Cale Nema14 (Autodesk Fusion 360 design; units mm, degrees)
Autodesk Fusion 360 part; units mm, degrees
sketch "Sketch1" plane through (0, 0, 0) normal (0, 0, 1) x (1, 0, 0)
  line L0 (24, 0) -> (24, 11) construction
  line L1 (-24, 11) -> (-24, 0) construction
  arc A0 (20.9184, 45.8497) -> (-20.9184, 45.8497) centre (0, 44) ccw construction
  line L2 (24, 11) -> (-24, 11) construction
  line L3 (-24, 0) -> (24, 0) construction
  line L4 (0, 44) -> (0, 11) construction
  line L5 (-24.1506, 0) -> (-24.1506, 11)
  line L6 (24.1506, 0) -> (24.1506, 11)
  line L7 (-23.1779, 22) -> (23.1779, 22)
  line L8 (-23.1779, 22) -> (-24.1506, 11)
  line L9 (24.1506, 11) -> (23.1779, 22)
  line L10 (24, 11) -> (20.9184, 45.8497) construction
  line L11 (-24, 11) -> (-20.9184, 45.8497) construction
  line L12 (-24.1506, 0) -> (24.1506, 0)
  line L13 (24, 0) -> (27, 0)
  line L14 (27, 0) -> (27, 22)
  line L15 (23.1779, 22) -> (27, 22)
  line L16 (-23.1779, 22) -> (-27, 22)
  line L17 (-27, 22) -> (-27, 0)
  line L18 (-27, 0) -> (-24, 0)
  dimension "d1" = 48
  dimension "d2" = 11
  dimension "d3" = 21
  dimension "d5" = 33
  dimension "d6" = 11
  dimension "d8" = 11
  dimension "d9" = 11
  dimension "d10" = 11
  dimension "d12" = 0.15
  dimension "d13" = 0.15
  dimension "d14" = 3
  dimension "d15" = 3
  constraint perpendicular L0 L3
  constraint perpendicular L0 L2
  constraint perpendicular L1 L2
  constraint coincident A0.centre L4.start
  constraint midpoint L2 L4.end
  constraint perpendicular L2 L4
  constraint horizontal L3
  constraint coincident origin L3
  constraint midpoint origin L3
  constraint perpendicular L3 L5
  constraint perpendicular L2 L6
  constraint perpendicular L4 L7
  constraint tangent A0 L10
  constraint tangent A0 L11
  constraint parallel L8 L11
  constraint parallel L9 L10
  constraint horizontal L12
  constraint perpendicular L6 L13
  constraint perpendicular L13 L14
  constraint perpendicular L16 L17
  constraint horizontal L18
  constraint horizontal L15
  constraint horizontal L16
  measures "d1" distance of L0.start L1.end
  measures "d2" distance of L1.start L1.end
  measures "d3" radius of A0
  measures "d5" distance of A0.centre L4.end
  measures "d6" distance of L5.end L7
  measures "d8" distance of L5.start L5.end
  measures "d9" distance of L6.start L6.end
  measures "d10" distance of L2 L7
  measures "d12" distance of L7.start L11
  measures "d13" distance of L7.end L10
  measures "d14" distance of L1.end L17.end
  measures "d15" distance of L0.start L13.end
extrude "Extrude1" add sketch "Sketch1" along normal blind 3 contours L5 L6 L7 L8 L9 L12 L13 L18
extrude "Extrude2" add sketch "Sketch1" along normal blind 20 contours L5 L8 L16 L17 L18 | L6 L9 L13 L14 L15
ref_plane "WorkPlane1" through (-24.1506, 11, 20) normal (0, -1, 0) x (1, 0, 0)
sketch "Sketch2" plane through (0, 11, 0) normal (0, -1, 0) x (1, 0, 0)
  line L0 (-27, 0) -> (27, 0)
  line L1 (27, 0) -> (27, 20)
  line L2 (27, 20) -> (24.1506, 20)
  line L3 (24.1506, 20) -> (24.1506, 3)
  line L4 (24.1506, 3) -> (-24.1506, 3)
  line L5 (-24.1506, 3) -> (-24.1506, 20)
  line L6 (-24.1506, 20) -> (-27, 20)
  line L7 (-27, 20) -> (-27, 0)
  line L8 (-27, 20) -> (27, 20)
  line L9 (27, 20) -> (27, 11.4)
  line L10 (27, 11.4) -> (-27, 11.4)
  line L11 (-27, 11.4) -> (-27, 20)
  dimension "d21" = 8.4
  constraint horizontal L8
  constraint vertical L9
  constraint horizontal L10
  constraint vertical L11
  constraint coincident L1 L9.end
  constraint coincident L6.end L7.start
  measures "d21" vertical distance of L4.end L10.end
extrude "Extrude3" add sketch "Sketch2" against normal blind 11 contours L3 L5 L8 L10
sketch "Sketch5" plane through (0, 11, 0) normal (0, -1, 0) x (1, 0, 0)
  line L0 (24.1506, 20) -> (-24.1506, 20)
  line L1 (-24.1506, 20) -> (-24.1506, 11.4)
  line L2 (-24.1506, 11.4) -> (24.1506, 11.4)
  line L3 (24.1506, 11.4) -> (24.1506, 20)
  line L4 (0, 0) -> (0, 20) construction
  line L5 (17.1, 11.4) -> (-17.1, 11.4)
  line L6 (-17.1, 11.4) -> (-17.1, 20)
  line L7 (-17.1, 20) -> (17.1, 20)
  line L8 (17.1, 20) -> (17.1, 11.4)
  line L9 (17.1, 11.4) -> (-17.1, 20) construction
  line L10 (-17.1, 11.4) -> (17.1, 20) construction
  point P0 (0, 15.7)
  dimension "d26" = 34.2
  constraint coincident L4.start origin
  constraint midpoint L0 L4.end
  constraint perpendicular L5 L6
  constraint parallel L5 L7
  constraint parallel L6 L8
  constraint horizontal L5
  constraint coincident L2 L5.start
  constraint coincident L9 P0
  constraint coincident L10 P0
  constraint coincident L4 P0
  constraint coincident L0 L6.end
  measures "d26" distance of L6 L8
extrude "Extrude4" cut sketch "Sketch5" against normal through all contours L0 L2 L5 L6 L7 L8
